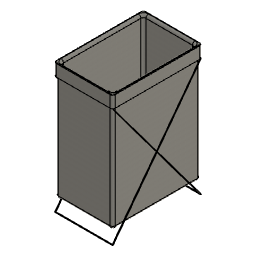
rgiro_astro_laundry_bag (Autodesk Fusion 360 design; units mm, degrees)
Autodesk Fusion 360 part; units mm, degrees
sketch "Sketch1" plane through (0, 0, 0) normal (0, 0, 1) x (1, 0, 0)
  line L0 (-115, -175) -> (115, -175)
  line L1 (115, -175) -> (115, 175)
  line L2 (115, 175) -> (-115, 175)
  line L3 (-115, 175) -> (-115, -175)
  line L4 (-115, -175) -> (115, 175) construction
  line L5 (115, -175) -> (-115, 175) construction
  dimension "d1" = 350
  dimension "d2" = 230
  constraint perpendicular L0 L1
  constraint parallel L0 L2
  constraint parallel L1 L3
  constraint horizontal L0
  constraint coincident L4 origin
  constraint coincident L5 origin
  measures "d1" distance of L0.start L2.end
  measures "d2" distance of L1.end L2.end
extrude "Extrude1" add sketch "Sketch1" along normal blind 510 makes body 1
sketch "Sketch2" plane through (0, 0, 0) normal (0, 0, -1) x (1, 0, 0)
  line L0 (-115, 175) -> (-115, -175)
  line L1 (-115, -175) -> (115, -175)
  line L2 (115, -175) -> (115, 175)
  line L3 (115, 175) -> (-115, 175)
  line L4 (-111, -171) -> (111, -171)
  line L5 (111, -171) -> (111, 171)
  line L6 (111, 171) -> (-111, 171)
  line L7 (-111, 171) -> (-111, -171)
  dimension "d5" = -4
extrude "Extrude2" cut sketch "Sketch2" against normal blind 460 bodies 1
sketch "Sketch3" plane through (0, -171, 0) normal (0, -1, 0) x (1, 0, 0)
  line L0 (-111, 0) -> (111, 0)
  line L1 (111, 0) -> (111, 460)
  line L2 (111, 460) -> (-111, 460)
  line L3 (-111, 460) -> (-111, 0)
  line L4 (-111, 0) -> (111, 0)
  line L5 (111, 0) -> (111, 50)
  line L6 (111, 50) -> (-111, 50)
  line L7 (-111, 50) -> (-111, 0)
  dimension "d8" = 50
  constraint horizontal L4
  constraint vertical L5
  constraint horizontal L6
  constraint vertical L7
  constraint coincident L1 L5.end
  constraint coincident L0.start L3.end
  measures "d8" distance of L0.start L6.end
extrude "Extrude3" cut sketch "Sketch3" against normal up to surface (342 mm away) contours L0 L1 L3 L4 L5 L6 L7 bodies 1
sketch "Sketch4" plane through (0, 0, 510) normal (0, 0, 1) x (-1, 0, 0)
  line L0 (115, -175) -> (115, 175)
  line L1 (115, 175) -> (-115, 175)
  line L2 (-115, 175) -> (-115, -175)
  line L3 (-115, -175) -> (115, -175)
  line L4 (101, 161) -> (-101, 161)
  line L5 (-101, 161) -> (-101, -161)
  line L6 (-101, -161) -> (101, -161)
  line L7 (101, -161) -> (101, 161)
  dimension "d11" = -14
extrude "Extrude4" cut sketch "Sketch4" against normal blind 450 contours L4 L5 L6 L7 bodies 1
sketch "Sketch7" plane through (0, 0, 0) normal (0, 0, 1) x (1, 0, 0)
  line L0 (-111, 171) -> (111, 171)
  line L1 (111, 171) -> (111, -171)
  line L2 (111, -171) -> (-111, -171)
  line L3 (-111, -171) -> (-111, 171)
  line L4 (111, 171) -> (-111, 171)
  line L5 (-111, 171) -> (-111, 173)
  line L6 (-111, 173) -> (111, 173)
  line L7 (111, 173) -> (111, 171)
  line L8 (-111, -171) -> (111, -171)
  line L9 (111, -171) -> (111, -173)
  line L10 (111, -173) -> (-111, -173)
  line L11 (-111, -173) -> (-111, -171)
  dimension "d18" = 2
  dimension "d19" = 2
  constraint horizontal L4
  constraint vertical L5
  constraint horizontal L6
  constraint vertical L7
  constraint coincident L0.end L1.start
  constraint horizontal L8
  constraint vertical L9
  constraint horizontal L10
  constraint vertical L11
  constraint coincident L2.end L3.start
  measures "d18" distance of L2.end L10.end
  measures "d19" distance of L0.end L6.end
extrude "Extrude7" add sketch "Sketch7" along normal blind 2 separate body contours L0 L4 L5 L6 L7 | L2 L8 L9 L10 L11 makes body 2 at (-37, 171, 0.6667) makes body 3 at (-37, -171.6667, 0)
sketch "Sketch8" plane through (-111, 0, 0) normal (-1, 0, 0) x (0, -1, 0)
  line L0 (-173, 0) -> (-171, 0)
  line L1 (-171, 0) -> (-171, 2)
  line L2 (-171, 2) -> (-173, 2)
  line L3 (-173, 2) -> (-173, 0)
  line L4 (-173, 2) -> (170, 460)
  line L5 (-171, 0) -> (172, 460)
  line L6 (170, 460) -> (172, 460)
  line L7 (173, 2) -> (-171, 460)
  line L8 (-171, 460) -> (-173, 460)
  line L9 (-173, 460) -> (171, 0)
  line L10 (171, 0) -> (173, 0)
  line L11 (173, 0) -> (173, 2)
  line L12 (-173, 2) -> (-173, 0)
  dimension "d22" = 2
  constraint coincident L2.end L3.start
  constraint coincident L0.end L1.start
  constraint horizontal L6
  constraint horizontal L8
  constraint parallel L8 L10
  constraint perpendicular L10 L11
  constraint coincident L0.start L3.end
  measures "d22" distance of L4.end L5.end
extrude "Extrude8" add sketch "Sketch8" along normal blind 2 separate body makes body 4
pattern_linear "R-Pattern1" count 2 spacing 224 along (1, 0, 0) of bodies 4 makes body 5
fillet "Fillet2" radius 10 5 faces at (101, -53.6667, 360) (-33.6667, -161, 210) (33.6667, -53.6667, 60) (-101, 53.6667, 360) (33.6667, 161, 210) on bodies 1
fillet "Fillet4" radius 10 4 edges at (-115, -175, 485) (115, -175, 485) (115, 175, 485) (-115, 175, 485) on bodies 1
fillet "Fillet5" radius 10 4 edges at (111, -171, 255) (111, 171, 255) (-111, -171, 255) (-111, 171, 255) 1 faces at (37, -57, 50) on bodies 1
fillet "Fillet6" radius 2 8 faces at (35, 175, 476.6667) (-114.8193, 166.8925, 476.6667) (-115, 55, 476.6667) (-114.8193, -166.8925, 476.6667) (-35, -175, 476.6667) (114.7181, -167.3576, 476.6667) (115, -55, 476.6667) (114.7181, 167.3576, 476.6667) on bodies 1
